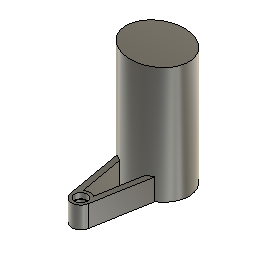
Throttle handle 1 (Autodesk Fusion 360 design; units mm, degrees)
Autodesk Fusion 360 part; units mm, degrees
sketch "Sketch1" plane through (0, 0, 0) normal (0, 0, 1) x (1, 0, 0)
  circle A0 centre (0, -26.6945) radius 3.075
  circle A1 centre (0, -26.6945) radius 5.075
  ellipse E0 centre (0, 15.9768) end of major axis (17.5, 15.9768) minor radius 15
  line L0 (-17.5, 15.9768) -> (17.5, 15.9768) construction
  line L1 (0, 0.9768) -> (0, 30.9768) construction
  line L2 (-4.9979, -27.5758) -> (-10.5694, 4.0217)
  line L3 (4.9979, -27.5758) -> (10.5694, 4.0217)
  line L4 (-2.8477, -22.4938) -> (-7.222, 2.3137)
  line L5 (7.2219, 2.3137) -> (2.8477, -22.4938)
  dimension "d1" = 6.15
  dimension "d2" = 2
  dimension "d3" = 35
  dimension "d4" = 30
  dimension "d5" = 10
  dimension "d6" = 10
  dimension "d7" = 3
  dimension "d8" = 3
  constraint coincident E0 L0.start
  constraint coincident E0 L0.end
  constraint coincident E0 L1.start
  constraint coincident E0 L1.end
  constraint horizontal L0
  constraint coincident A1 L2.start
  constraint coincident E0 L2.end
  constraint tangent A1 L2
  constraint coincident A1 L3.start
  constraint coincident E0 L3.end
  constraint tangent A1 L3
  constraint coincident A1 L4.start
  constraint coincident E0 L4.end
  constraint parallel L2 L4
  constraint coincident E0 L5.start
  constraint coincident A1 L5.end
  constraint parallel L3 L5
  measures "d1" diameter of A0
  measures "d3" distance of E0
  measures "d5" angle of L1 L2
  measures "d6" angle of L1 L3
  measures "d7" distance of L2 L4
  measures "d8" distance of L3 L5
extrude "Extrude1" add sketch "Sketch1" along normal blind 12 contours A1 | A1 E0 L3 L5 | A1 E0 L2 L4 | E0 makes body 1
sketch "Sketch2" plane through (0, 0, 12) normal (0, 0, 1) x (-1, 0, 0)
  circle A0 centre (0, 26.6945) radius 3.075
  ellipse E0 centre (0, -15.9768) end of major axis (-17.5, -15.9768) minor radius 15 (7.222, -2.3137) -> (-7.2219, -2.3137) ccw
  line L0 (-7.2219, -2.3137) -> (-2.8477, 22.4938)
  arc A1 (-2.8477, 22.4938) -> (2.8477, 22.4938) centre (0, 26.6945) ccw
  line L1 (2.8477, 22.4938) -> (7.222, -2.3137)
  arc A2 (4.9979, 27.5758) -> (-4.9979, 27.5758) centre (0, 26.6945) ccw
  line L2 (-4.9979, 27.5758) -> (-10.5694, -4.0217)
  ellipse E1 centre (0, -15.9768) end of major axis (-17.5, -15.9768) minor radius 15 (-10.5694, -4.0217) -> (10.5694, -4.0217) ccw
  line L3 (10.5694, -4.0217) -> (4.9979, 27.5758)
  circle A3 centre (0, 26.6945) radius 3.5
  dimension "d11" = 7
  constraint concentric A0 A3
  measures "d11" diameter of A3
extrude "Extrude2" cut sketch "Sketch2" against normal blind 3 contours A3 bodies 1
extrude "Extrude3" add sketch "Sketch1" against normal blind 53 separate body contours E0 makes body 2
move_body "Move1" bodies 2 to x (1, 0, 0) y (0, 1, 0) z (0, 0, 1) at (0, 0, 65)
combine "Combine1" operation add target body 1 tool bodies 2
equation "d14 = -( 65 mm - 12 mm )"
